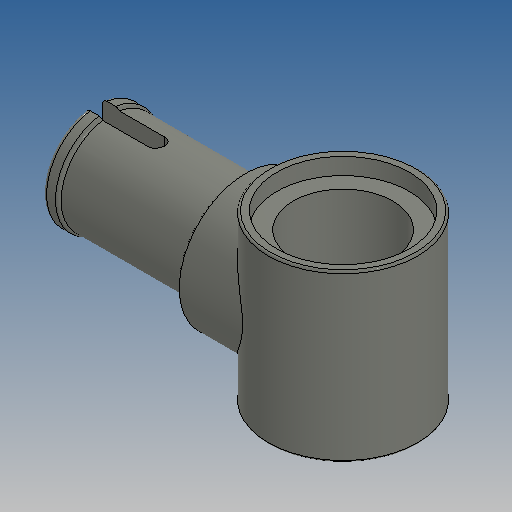
# Autodesk Inventor part: 15100-DkBluishGray
Saved by Autodesk Inventor 2025 (Build 290162010, 162A)
## iProperties
Created: 2012-03-21
Part Number: 15100-DkBluishGray
Document SubType Name: Modeling
Designer: D. Kohfeld
Density: 1.06 g/cm^3
Material: ABS Plastic
Mass: 0.284668 g
Surface Area: 5.85338 cm^2
Volume: 0.268555 cm^3
Appearance: DkBluishGray
Author: D. Kohfeld
Autodesk Inventor part; units mm, degrees
ref_plane "YZ Plane" through (0, 0, 0) normal (1, 0, 0) x (0, 1, 0)
ref_plane "XZ Plane" through (0, 0, 0) normal (0, 1, 0) x (-1, 0, 0)
ref_plane "XY Plane" through (0, 0, 0) normal (0, 0, 1) x (1, 0, 0)
sketch "Sketch1" plane through (0, 0, 0) normal (0, 0, 1) x (1, 0, 0)
  circle A0 centre (0, 0) radius 3.2
  circle A1 centre (0, 0) radius 2.4
  circle A2 centre (0, 0) radius 3.6
  dimension "d48" = 7.2
  dimension "d49" = 6.4
  dimension "d50" = 4.8
  constraints: 3 centre point, 3 coincident
  measures "d48" diameter of A2
  measures "d49" diameter of A0
  measures "d50" diameter of A1
extrude "Extrusion1" add sketch "Sketch1" along normal mid plane 8 contours A0 | A2
sketch "Sketch6" plane through (0, 0, 4) normal (0, 0, 1) x (1, 0, 0)
  circle A0 centre (0, 0) radius 2.4 projected
  circle A1 centre (0, 0) radius 3.2 projected
extrude "Extrusion7" cut sketch "Sketch6" against normal blind 0.8
mirror "Mirror1" about plane through (0, 0, 0) normal (0, 0, 1) of "Extrusion7"
sketch "Sketch7" plane through (0, 0, 0) normal (0, 0, 1) x (1, 0, 0)
  circle A0 centre (0, 0) radius 3.6 projected
  line L0 (-3.2249, 1.6) -> (-12, 1.6)
  line L1 (-12, 1.6) -> (-12, 2.5)
  line L2 (-12, 2.5) -> (-11.2, 2.5)
  line L3 (-11.2, 2.5) -> (-11.2, 2.4)
  line L4 (-11.2, 2.4) -> (-4.8, 2.4)
  line L5 (-4.8, 2.4) -> (-4.8, 3.2)
  line L6 (-4.8, 3.2) -> (-3.2249, 3.2)
  line L7 (-3.2249, 3.2) -> (-3.2249, 1.6)
  line L8 (-12, 0.4) -> (-12, -0.4)
  line L9 (-12, -0.4) -> (-9, -0.4)
  arc A1 (-9, -0.4) -> (-9, 0.4) centre (-9, 0) ccw
  line L10 (-9, 0.4) -> (-12, 0.4)
  line L11 (-15.12, 0) -> (6.72, 0) projected
  dimension "d53" = 7.2
  dimension "d54" = 0.8
  dimension "d55" = 4.8
  dimension "d58" = 3.4
  dimension "d59" = 0.8
  dimension "d62" = 6.4
  dimension "d63" = 3.2
  dimension "d64" = 5
  dimension "d65" = 4.8
  constraints: 22 end point, 3 vertical, 2 parallel, 2 point on circle, 2 tangent, 1 centre point, 1 horizontal alignment, 1 perpendicular, 1 vertical alignment, 2 other
  measures "d53" distance between parallel lines of L1 L5
  measures "d54" distance of L1.end L2.end
  measures "d55" distance from line of L5 point (0, 0)
  measures "d59" distance between parallel lines of L10 L9
  measures "d62" diameter of L6 L11
  measures "d63" diameter of L0 L11
  measures "d64" diameter of L2 L11
  measures "d65" diameter of L4 L11
revolve "Revolution1" add sketch "Sketch7" angle 360 about axis through (-10, 0, 0) along (1, 0, 0) contours L0 L1 L2 L3 L4 L5 L6 L7
sketch "Sketch8" plane through (-3.2249, 0, 0) normal (1, 0, 0) x (0, 0, -1)
  line L0 (0, -1.6) -> (2.7713, -1.6) projected
  line L1 (-2.7713, -1.6) -> (0, -1.6) projected
  arc A0 (-2.7713, -1.6) -> (2.7713, -1.6) centre (0, 0) ccw projected
  line L2 (2.7713, 1.6) -> (0, 1.6) projected
  arc A1 (2.7713, 1.6) -> (-2.7713, 1.6) centre (0, 0) ccw projected
  line L3 (0, 1.6) -> (-2.7713, 1.6) projected
extrude "Extrusion9" add sketch "Sketch8" along normal up to next
extrude "Extrusion10" cut sketch "Sketch7" along normal through all both and the other way through all contours L10 A1 L11 L8 | L11 A1 L9 L8
fillet "Fillet2" radius 0.1 3 edges at (-3.6, 0, 4) (-4.8, -3.2, 0) (-3.6, 0, -4)
fillet "Fillet2" radius 0.2 4 edges at (-12, -2.5, 0) (-11.2, -2.5, 0) (-12, 2.5, 0) (-11.2, 2.5, 0)
equation "\"lf\" = 0.1"
equation "\"pinf\" = 0.2"
body "Solid1"
